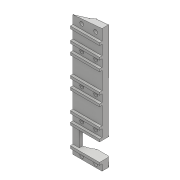
# Autodesk Inventor part: Hand - Distal Bridge
Saved by Autodesk Inventor 2017 (Build 210142000, 142)
## iProperties
Created: 2016-09-27
Part Number: Hand - Distal Bridge
Material: Generic
Document SubType Name: Modeling
Designer: cmcdona
Density: 1 g/cm^3
Appearance: Default
Author: cmcdona
Autodesk Inventor part; units mm, degrees
ref_plane "YZ Plane" through (0, 0, 0) normal (1, 0, 0) x (0, 1, 0)
ref_plane "XZ Plane" through (0, 0, 0) normal (0, 1, 0) x (-1, 0, 0)
sketch "Sketch1" plane through (0, 0, 0) normal (0, 0, 1) x (1, 0, 0)
  line L0 (0, 0) -> (114, 0)
  arc A0 (114, 0) -> (114, 18) centre (114, 9) ccw
  arc A1 (0, 21) -> (0, 0) centre (0, 10.5) ccw
  line L1 (0, 21) -> (20.7846, 18)
  line L2 (20.7846, 18) -> (114, 18)
  dimension "d0" = 114
  dimension "d1" = 18
  dimension "d2" = 9
  dimension "d3" = 21
  dimension "d4" = 10.5
  dimension "d5" = 21
  constraints: 6 end point, 4 point on circle, 2 centre point, 2 horizontal
  measures "d0" distance of L0.start L0.end
  measures "d1" distance of L0.end L2.end
  measures "d2" radius of A0
  measures "d3" distance of L0.start L1.start
  measures "d4" radius of A1
  measures "d5" distance of L1.start L1.end
extrude "Extrusion1" add sketch "Sketch1" against normal blind 100
sketch "Sketch6" plane through (0, 0, 0) normal (0, 0, 1) x (1, 0, 0)
  line L0 (20.7846, 18) -> (114, 18) projected
  line L1 (91, 18) -> (114, 18)
  line L2 (114, 18) -> (114, 24)
  line L3 (114, 24) -> (104, 24)
  line L4 (104, 24) -> (100.5359, 22)
  line L5 (100.5359, 22) -> (91, 19)
  line L6 (91, 19) -> (91, 18)
  point P0 (0, 0)
  dimension "d37" = 23
  dimension "d38" = 6
  dimension "d39" = 10
  dimension "d40" = 4
  dimension "d41" = 150
  constraints: 12 end point, 2 perpendicular, 1 collinear, 1 parallel
  measures "d37" distance of L1.start L0.end
  measures "d38" distance of L0.end L2.end
  measures "d39" distance of L2.end L3.end
  measures "d40" distance of L3.end L4.end
  measures "d41" angle of L4 L3
extrude "Extrusion6" add sketch "Sketch6" against normal blind 100
sketch "Sketch7" plane through (0, 0, 0) normal (0, -1, 0) x (1, 0, 0)
  line L0 (0, 0) -> (-10.5, 0) projected
  line L1 (-10.5, 0) -> (-10.5, -8)
  line L2 (-10.5, 0) -> (-10.5, -100) projected
  line L3 (-10.5, -8) -> (49, -8)
  line L4 (49, -8) -> (140.4404, 0)
  line L5 (140.4404, 0) -> (-10.5, 0)
  dimension "d44" = 8
  dimension "d45" = 59.5
  dimension "d46" = 90
  dimension "d47" = 175
  constraints: 8 end point, 1 parallel, 1 perpendicular, 1 point on line
  measures "d44" distance of L0.end L1.end
  measures "d45" distance of L1.end L3.end
  measures "d46" angle of L3 L1
  measures "d47" angle of L4 L3
extrude "Extrusion7" cut sketch "Sketch7" against normal through all
ref_plane "Work Plane2" through (0, 0, 0) normal (0, 0, 1) x (1, 0, 0)
sketch "Sketch8" plane through (0, 0, 0) normal (0, 0, 1) x (1, 0, 0)
  line L0 (-10.5, 0) -> (70, 0)
  line L1 (70, 0) -> (70, 21)
  line L2 (70, 21) -> (-10.5, 21)
  line L3 (-10.5, 21) -> (-10.5, 0)
  line L4 (70, 0) -> (125, 0)
  line L5 (125, 0) -> (125, 18)
  line L6 (125, 18) -> (70, 18)
  line L7 (70, 18) -> (70, 0)
  point P0 (0, 0)
  dimension "d51" = 80.5
  dimension "d52" = 21
  dimension "d53" = 55
  dimension "d54" = 18
  constraints: 16 end point, 4 parallel, 2 horizontal, 2 perpendicular
  measures "d51" distance of L2.end L1.end
  measures "d52" distance of L1.end L0.end
  measures "d53" distance of L6.end L5.end
  measures "d54" distance of L5.end L4.end
extrude "Extrusion8" cut sketch "Sketch8" against normal blind 100
sketch "Sketch9" plane through (91, 18, -100) normal (0, -1, 0) x (1, 0, 0)
  line L0 (23, 97.6868) -> (23, 0) projected
  line L1 (0, 5) -> (23, 5)
  line L2 (23, 5) -> (23, 7)
  line L3 (23, 7) -> (0, 7)
  line L4 (0, 7) -> (0, 5)
  line L5 (0, 95.6745) -> (0, 0) projected
  line L6 (0, 23) -> (23, 23)
  line L7 (23, 23) -> (23, 21)
  line L8 (23, 21) -> (0, 21)
  line L9 (0, 21) -> (0, 23)
  line L10 (0, 29) -> (23, 29)
  line L11 (23, 29) -> (23, 31)
  line L12 (23, 31) -> (0, 31)
  line L13 (0, 31) -> (0, 29)
  line L14 (0, 47) -> (23, 47)
  line L15 (23, 47) -> (23, 45)
  line L16 (23, 45) -> (0, 45)
  line L17 (0, 45) -> (0, 47)
  line L18 (0, 53) -> (23, 53)
  line L19 (23, 53) -> (23, 55)
  line L20 (23, 55) -> (0, 55)
  line L21 (0, 55) -> (0, 53)
  line L22 (0, 71) -> (23, 71)
  line L23 (23, 71) -> (23, 69)
  line L24 (23, 69) -> (0, 69)
  line L25 (0, 69) -> (0, 71)
  line L26 (0, 77) -> (23, 77)
  line L27 (23, 77) -> (23, 79)
  line L28 (23, 79) -> (0, 79)
  line L29 (0, 79) -> (0, 77)
  line L30 (0, 89) -> (23, 89)
  line L31 (23, 89) -> (23, 87)
  line L32 (23, 87) -> (0, 87)
  line L33 (0, 87) -> (0, 89)
  point P0 (-91, 100)
  dimension "d57" = 2
  dimension "d58" = 2
  dimension "d59" = 2
  dimension "d60" = 2
  dimension "d61" = 2
  dimension "d62" = 2
  dimension "d63" = 2
  dimension "d64" = 2
  constraints: 64 end point, 16 parallel, 8 horizontal, 8 perpendicular, 1 point on line, 16 other
  measures "d57" distance of L2.end L1.end
  measures "d58" distance of L6.end L7.end
  measures "d59" distance of L11.end L10.end
  measures "d60" distance of L14.end L15.end
  measures "d61" distance of L19.end L18.end
  measures "d62" distance of L22.end L23.end
  measures "d63" distance of L27.end L26.end
  measures "d64" distance of L30.end L31.end
extrude "Extrusion9" add sketch "Sketch9" along normal blind 2 contours L0 L32 L5 L30 | L0 L26 L5 L28 | L0 L24 L5 L22 | L0 L18 L5 L20 | L0 L16 L5 L14 | L0 L10 L5 L12 | L0 L8 L5 L6 | L0 L1 L4 L3
sketch "Sketch10" plane through (91, 18, -11) normal (0, -1, 0) x (1, 0, 0)
  circle A0 centre (18, 4) radius 1.5
  circle A1 centre (7, 4) radius 1.5
  circle A2 centre (7, -15) radius 1.5
  circle A3 centre (7, -39) radius 1.5
  circle A4 centre (7, -63) radius 1.5
  circle A5 centre (7, -86.5) radius 1.5
  circle A6 centre (18, -15) radius 1.5
  circle A7 centre (18, -39) radius 1.5
  circle A8 centre (18, -63) radius 1.5
  circle A9 centre (18, -86.5) radius 1.5
  point P0 (-91, 11)
  dimension "d67" = 3
  dimension "d68" = 3
  dimension "d69" = 3
  dimension "d70" = 3
  dimension "d71" = 3
  dimension "d72" = 3
  dimension "d73" = 3
  dimension "d74" = 3
  dimension "d75" = 3
  dimension "d76" = 3
  constraints: 10 centre point
  measures "d67" diameter of A0
  measures "d68" diameter of A1
  measures "d69" diameter of A2
  measures "d70" diameter of A3
  measures "d71" diameter of A4
  measures "d72" diameter of A5
  measures "d73" diameter of A6
  measures "d74" diameter of A7
  measures "d75" diameter of A8
  measures "d76" diameter of A9
extrude "Extrusion10" cut sketch "Sketch10" against normal through all
fillet "Fillet1" radius 1 7 edges at (114, 24, -51.1566) (109, 24, -100) (102.2679, 23, -100) (95.7679, 20.5, -100) (109, 24, -2.7507) (102.2679, 23, -3.3397) (95.7679, 20.5, -3.9083)
sketch "Sketch12" plane through (91, 18, -93) normal (0, 0, 1) x (1, 0, 0)
  line L0 (23, 0) -> (5, 0)
  line L1 (5, 0) -> (5, 6)
  line L2 (5, 6) -> (23, 6)
  line L3 (23, 6) -> (23, 0)
  point P0 (-91, -18)
  dimension "d84" = 18
  dimension "d85" = 6
  constraints: 8 end point, 2 parallel, 1 horizontal, 1 perpendicular
  measures "d84" distance of L1.end L2.end
  measures "d85" distance of L0.end L1.end
extrude "Extrusion12" cut sketch "Sketch12" along normal blind 14
body "Solid1"
